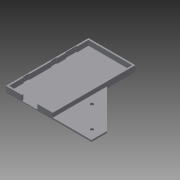
# Autodesk Inventor part: Phone_Holder
Saved by Autodesk Inventor 2013 (Build 170138000, 138)
## iProperties
Created: 2015-03-29
Part Number: Phone_Holder
Material: Generic
Document SubType Name: Modeling
Designer: Pat
Density: 1 g/cm^3
Author: Pat
Autodesk Inventor part; units mm, degrees
ref_plane "YZ Plane" through (0, 0, 0) normal (1, 0, 0) x (0, 1, 0)
ref_plane "XZ Plane" through (0, 0, 0) normal (0, 1, 0) x (-1, 0, 0)
ref_plane "XY Plane" through (0, 0, 0) normal (0, 0, 1) x (1, 0, 0)
sketch "Sketch1" plane through (0, 0, 0) normal (0, 1, 0) x (-1, 0, 0)
  line L0 (-128.4561, -59.0678) -> (-200.0841, -59.0678)
  line L1 (-200.0841, -59.0678) -> (-200.0841, 71.2342)
  line L2 (-200.0841, 71.2342) -> (-128.4561, 71.2342)
  line L3 (-128.4561, 71.2342) -> (-128.4561, 47.3963)
  line L4 (-128.4561, 47.3963) -> (-127.1861, 47.3963)
  line L5 (-127.1861, 47.3963) -> (-127.1861, 37.9983)
  line L6 (-127.1861, 37.9983) -> (-128.4561, 37.9983)
  line L7 (-128.4561, 37.9983) -> (-128.4561, 1.9684)
  line L8 (-128.4561, 1.9684) -> (-127.1861, 1.9684)
  line L9 (-127.1861, 1.9684) -> (-127.1861, -7.4296)
  line L10 (-127.1861, -7.4296) -> (-128.4561, -7.4296)
  line L11 (-128.4561, -7.4296) -> (-128.4561, -21.9584)
  line L12 (-128.4561, -21.9584) -> (-127.1861, -21.9584)
  line L13 (-127.1861, -21.9584) -> (-127.1861, -40.2464)
  line L14 (-127.1861, -40.2464) -> (-128.4561, -40.2464)
  line L15 (-128.4561, -40.2464) -> (-128.4561, -59.0678)
  line L16 (-202.6241, 73.7742) -> (-125.9161, 73.7742)
  line L17 (-125.9161, 73.7742) -> (-125.9161, -61.6078)
  line L18 (-125.9161, -61.6078) -> (-202.6241, -61.6078)
  line L19 (-202.6241, -61.6078) -> (-202.6241, 73.7742)
  circle A0 centre (-164.6511, -28.5878) radius 4.9213 construction
  line L20 (-202.6241, 73.7742) -> (-266.1241, 73.7742)
  line L21 (-164.6511, 373.4543) -> (-228.1511, 373.4543) construction
  line L22 (-228.1511, 373.4543) -> (-228.1511, 106.7543) construction
  line L23 (-228.1511, 106.7543) -> (-299.9932, 34.9122) construction
  line L24 (-299.9932, 34.9122) -> (-668.2932, 34.9122) construction
  line L25 (-668.2932, 34.9122) -> (-668.2932, -28.5878) construction
  line L26 (-668.2932, -28.5878) -> (-223.7932, -28.5878) construction
  line L27 (-223.7932, -28.5878) -> (-164.6511, 30.5543) construction
  line L28 (-164.6511, 30.5543) -> (-164.6511, 373.4543) construction
  line L29 (-264.0722, 70.8332) -> (-194.2222, 0.9832) construction
  line L30 (-164.6511, 30.5543) -> (-164.6511, -28.5878) construction
  line L31 (-164.6511, -28.5878) -> (-223.7932, -28.5878) construction
  circle A1 centre (-251.4998, 58.2609) radius 2.54
  circle A2 centre (-215.5788, 22.3399) radius 2.54
  line L32 (-266.1241, 73.7742) -> (-266.1241, 48.3742)
  line L33 (-266.1241, 48.3742) -> (-202.6241, -15.1258)
  line L34 (-177.3511, 73.7742) -> (-177.3511, 71.2342)
  line L35 (-151.9511, 73.7742) -> (-151.9511, 71.2342)
  point P0 (0, 0)
  dimension "d0" = 71.628
  dimension "d3" = 130.302
  dimension "d4" = 9.398
  dimension "d5" = 9.398
  dimension "d6" = 18.288
  dimension "d7" = 23.8379
  dimension "d8" = 36.0299
  dimension "d9" = 14.5288
  dimension "d10" = 1.27
  dimension "d11" = 2.54
  dimension "d12" = 2.54
  dimension "d13" = 2.54
  dimension "d14" = 2.54
  dimension "d15" = 9.8425
  dimension "d17" = 36.195
  dimension "d18" = 30.48
  dimension "d19" = 63.5
  dimension "d20" = 63.5
  dimension "d21" = 63.5
  dimension "d22" = 101.6
  dimension "d23" = 266.7
  dimension "d24" = 368.3
  dimension "d25" = 444.5
  dimension "d26" = 342.9
  dimension "d27" = 5.08
  dimension "d28" = 5.08
  dimension "d29" = 17.78
  dimension "d30" = 68.58
  dimension "d31" = 25.4
  dimension "d44" = 12.7
  dimension "d45" = 12.7
  constraints: 72 end point, 22 parallel, 9 perpendicular, 7 point on line, 6 collinear, 3 centre point, 2 horizontal, 2 midpoint, 1 coincident
  measures "d0" distance of L0.start L0.end
  measures "d3" distance of L0.end L1.end
  measures "d4" distance of L4.end L5.end
  measures "d5" distance of L8.end L9.end
  measures "d6" distance of L12.end L13.end
  measures "d7" distance of L2.end L3.end
  measures "d8" distance of L6.end L7.end
  measures "d9" distance of L10.end L11.end
  measures "d10" distance of L13.end L14.end
  measures "d11" horizontal distance of L16.end L2.end
  measures "d12" horizontal distance of L1.end L16.start
  measures "d13" horizontal distance of L2.end L16.end
  measures "d14" horizontal distance of L17.end L0.start
  measures "d15" diameter of A0
  measures "d17" horizontal distance of A0.centre L0.start
  measures "d18" vertical distance of L0.start A0.centre
  measures "d19" distance of L16.start L20.end
  measures "d20" distance of L21.start L21.end
  measures "d21" distance of L24.end L25.end
  measures "d22" distance of L22.end L23.end
  measures "d23" distance of L21.end L22.end
  measures "d24" distance of L23.end L24.end
  measures "d25" distance of L25.end L26.end
  measures "d26" distance of L27.end L21.start
  measures "d27" diameter of A1
  measures "d28" diameter of A2
  measures "d29" distance from line of L23 A1.centre
  measures "d30" distance from line of L23 A2.centre
  measures "d31" distance of L20.end L32.end
  measures "d44" distance between parallel lines of L28 L34
  measures "d45" distance between parallel lines of L28 L35
sketch "Sketch2" plane through (0, 0, 0) normal (0, 1, 0) x (-1, 0, 0)
  line L0 (-202.6241, -61.6078) -> (-202.6241, 73.7742)
  line L1 (-202.6241, 73.7742) -> (-266.1241, 73.7742)
  line L2 (-264.0722, 70.8332) -> (-194.2222, 0.9832) construction
  circle A0 centre (-251.4998, 58.2609) radius 2.54
  circle A1 centre (-215.5788, 22.3399) radius 2.54
  line L3 (-266.1241, 73.7742) -> (-266.1241, 48.3742)
  line L4 (-266.1241, 48.3742) -> (-202.6241, -15.1258)
  point P0 (0, 0)
  dimension "d32" = 63.5
  dimension "d33" = 5.08
  dimension "d34" = 5.08
  dimension "d35" = 25.4
  constraints: 10 end point, 3 point on line, 2 centre point, 1 parallel, 1 perpendicular
  measures "d32" distance of L1.start L1.end
  measures "d33" diameter of A0
  measures "d34" diameter of A1
  measures "d35" distance of L1.end L3.end
sketch "Sketch3" plane through (0, 0, 0) normal (0, 1, 0) x (-1, 0, 0)
  line L0 (-202.6241, 73.7742) -> (-125.9161, 73.7742)
  line L1 (-125.9161, 73.7742) -> (-125.9161, -61.6078)
  line L2 (-125.9161, -61.6078) -> (-202.6241, -61.6078)
  line L3 (-202.6241, -61.6078) -> (-202.6241, 73.7742)
  line L4 (-202.6241, 73.7742) -> (-266.1241, 73.7742)
  line L5 (-266.1241, 73.7742) -> (-266.1241, 48.3742)
  line L6 (-266.1241, 48.3742) -> (-202.6241, -15.1258)
  point P0 (0, 0)
  dimension "d36" = 63.5
  dimension "d37" = 25.4
  constraints: 14 end point, 2 parallel, 2 perpendicular, 1 horizontal, 1 point on line
  measures "d36" distance of L0.start L5.start
  measures "d37" distance of L5.start L5.end
extrude "Extrusion4" add sketch "Sketch1" along normal blind 9.525 contours L15 L14 L13 L12 L11 L10 L9 L8 L7 L6 L5 L4 L3 L2 L35 L16 L17 L18 L19 L34 L1 L0
extrude "Extrusion5" add sketch "Sketch2" along normal blind 2.54
extrude "Extrusion6" add sketch "Sketch3" along normal blind 1.27 contours L0 L1 L2 L3
body "Solid2"
